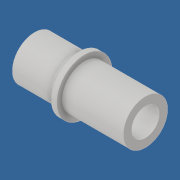
# Autodesk Inventor part: Lagerbuchse
Saved by Autodesk Inventor 2018 (Build 220112000, 112)
## iProperties
Created: 2018-10-09
Part Number: Lagerbuchse
Material: Generisch
Document SubType Name: Modeling
Designer: M.Knabel
Density: 1 g/cm^3
Appearance: Vorgabe
Author: M.Knabel
Autodesk Inventor part; units mm, degrees
ref_plane "YZ Plane" through (0, 0, 0) normal (1, 0, 0) x (0, 1, 0)
ref_plane "XZ Plane" through (0, 0, 0) normal (0, 1, 0) x (-1, 0, 0)
ref_plane "XY Plane" through (0, 0, 0) normal (0, 0, 1) x (1, 0, 0)
sketch "Skizze1" plane through (0, 0, 0) normal (0, 0, 1) x (1, 0, 0)
  line L0 (-4, 0) -> (24, 0) projected
  line L1 (0, -1) -> (0, 6) projected
  line L2 (0, 2.5) -> (20, 2.5)
  line L3 (20, 2.5) -> (20, 4)
  line L4 (20, 4) -> (9, 4)
  line L5 (9, 4) -> (9, 5)
  line L6 (9, 5) -> (8, 5)
  line L7 (8, 5) -> (8, 4)
  line L8 (8, 4) -> (0, 4)
  line L9 (0, 4) -> (0, 2.5)
  point P0 (0, 0)
  dimension "d0" = 10
  dimension "d1" = 8
  dimension "d2" = 8
  dimension "d3" = 11
  dimension "d4" = 5
  dimension "d5" = 20
  constraints: 16 end point, 5 perpendicular, 3 point on line, 1 collinear, 1 horizontal, 1 midpoint
  measures "d0" diameter of L6 L0
  measures "d1" diameter of L4 L0
  measures "d2" distance between parallel lines of L7 L1
  measures "d3" distance between parallel lines of L3 L5
  measures "d4" diameter of L2 L0
  measures "d5" distance between parallel lines of L3 L1
revolve "Umdrehung1" add sketch "Skizze1" angle 360 about axis through (-10, 0, 0) along (1, 0, 0)
fillet "Rundung1" radius 1.3 1 edges at (8, -4, 0)
